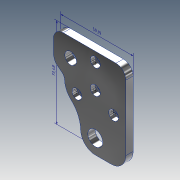
# Autodesk Inventor part: ZBaringBracket
Saved by Autodesk Inventor 2019 (Build 230136000, 136)
## iProperties
Created: 2018-10-14
Part Number: ZBaringBracket
Material: Aluminum 6061
Document SubType Name: Modeling
Designer: LillaHunden
Density: 2.7 g/cm^3
Appearance: Aluminum - Flat
Mass: 59.817 g
Surface Area: 75.5547 cm^2
Volume: 22.1545 cm^3
Author: LillaHunden
Autodesk Inventor part; units mm, degrees
ref_plane "YZ Plane" through (0, 0, 0) normal (1, 0, 0) x (0, 1, 0)
ref_plane "XZ Plane" through (0, 0, 0) normal (0, 1, 0) x (-1, 0, 0)
ref_plane "XY Plane" through (0, 0, 0) normal (0, 0, 1) x (1, 0, 0)
sketch "Sketch1" plane through (0, 0, 0) normal (0, 0, 1) x (1, 0, 0)
  line L0 (6, -5.5) -> (6, -7.5) construction
  line L1 (6, -7.5) -> (25, -7.5) construction
  line L2 (25, -7.5) -> (25, 7.5) construction
  line L3 (25, 7.5) -> (7.55, 7.5) construction
  line L4 (7.55, 7.5) -> (7.55, 2.5) construction
  line L5 (7.55, 2.5) -> (-7.55, 2.5) construction
  line L6 (-7.55, 2.5) -> (-7.55, 7.5) construction
  line L7 (-7.55, 7.5) -> (-25, 7.5) construction
  line L8 (-25, 7.5) -> (-25, -7.5) construction
  line L9 (-25, -7.5) -> (-6, -7.5) construction
  line L10 (-6, -7.5) -> (-6, -5.5) construction
  line L11 (-6, -5.5) -> (6, -5.5) construction
  line L12 (-7.45, 15.5) -> (7.55, 15.5) construction
  line L13 (-7.45, 2.5) -> (-7.45, 15.5) construction
  line L14 (7.55, 2.5) -> (-7.45, 2.5) construction
  line L15 (7.55, 2.5) -> (7.55, 15.5) construction
  line L16 (25, -7.5) -> (-34.185, -7.5)
  line L17 (-34.185, -7.5) -> (-34.185, 35.7282)
  line L18 (-34.185, 35.7282) -> (25, 35.7282)
  line L19 (25, 35.7282) -> (25, -7.5)
  circle A0 centre (15, 0) radius 1.621 projected
  circle A1 centre (-15, 0) radius 1.621 projected
  point P0 (0, 0)
  constraints: 8 end point, 2 parallel, 1 horizontal, 1 perpendicular, 1 point on line
extrude "Extrusion1" add sketch "Sketch1" along normal blind 6 contours L16 L17 L18 L19 | A0 | A1
sketch "Sketch8" plane through (0, 0, 6) normal (0, 0, 1) x (1, 0, 0)
  line L0 (-25, 7.5) -> (-25, -7.5) construction
  line L1 (-7.55, 7.5) -> (-25, 7.5) construction
  circle A0 centre (-20.1, 20.7) radius 5.5 construction
  line L2 (-34.185, -7.5) -> (-34.185, 35.7282) projected
  line L3 (-34.185, 14.1141) -> (-25, 0)
  line L4 (-25, -7.5) -> (-25, 0)
  line L5 (-34.185, 14.1141) -> (-34.185, 26.4425)
  line L6 (-34.185, 35.7282) -> (25, 35.7282) projected
  line L7 (-34.185, -7.5) -> (25, -7.5) projected
  point P0 (0, 0)
  constraints: 6 end point, 2 midpoint, 1 collinear, 1 point on line
extrude "Extrusion4" cut sketch "Sketch8" against normal through all
fillet "Fillet1" radius 3 1 edges at (-25, 0, 3)
fillet "Fillet2" radius 12 1 edges at (-34.185, 14.1141, 3)
fillet "Fillet4" radius 8 1 edges at (-34.185, 35.7282, 3)
fillet "Fillet5" radius 8 1 edges at (25, 35.7282, 3)
sketch "Sketch9" plane through (0, 0, 0) normal (0, 0, -1) x (-1, 0, 0)
  circle A0 centre (20.1, 20.7) radius 4.765
  arc A1 (21.2721, 23.6507) -> (18.4534, 23.4146) centre (20.1, 20.7) ccw projected
  point P0 (0, 0)
  dimension "d32" = 9.53
  constraints: 1 centre point
  measures "d32" diameter of A0
extrude "Extrusion5" cut sketch "Sketch9" against normal blind 3.3
sketch "Sketch10" plane through (-20.1, 20.7, 3.3) normal (0, 0, -1) x (-1, 0, 0)
  circle A0 centre (0, 0) radius 3.25
  point P0 (-20.1, -20.7)
  dimension "d35" = 6.5
  constraints: 1 centre point
  measures "d35" diameter of A0
extrude "Extrusion6" cut sketch "Sketch10" against normal through all
sketch "Sketch11" plane through (25, -7.5, 0) normal (0, -1, 0) x (1, 0, 0)
  line L0 (-50, 6) -> (-50, 0) projected
  line L1 (0, 0) -> (-50, 0) projected
  line L2 (0, 0) -> (0, 6) projected
  line L3 (-50, 6) -> (0, 6) projected
  point P0 (-25, 0)
extrude "Extrusion7" add sketch "Sketch11" along normal blind 30.25
sketch "Sketch12" plane through (0, 0, 6) normal (0, 0, 1) x (1, 0, 0)
  circle A0 centre (0.0605, -25.75) radius 6.1
  line L0 (25, -37.75) -> (-25, -37.75) projected
  point P0 (0, 0)
  dimension "d40" = 12.2
  dimension "d41" = 12
  constraints: 1 centre point
  measures "d40" diameter of A0
  measures "d41" distance from line of A0.centre L0
extrude "Extrusion8" cut sketch "Sketch12" against normal through all
fillet "Fillet6" radius 12 2 edges at (-25, -37.75, 3) (25, -37.75, 3)
sketch "Sketch13" plane through (0, 0, 6) normal (0, 0, 1) x (1, 0, 0)
  line L0 (-25, 5.4183) -> (-25, -8.3317) projected
  arc A0 (-34.185, 17.6749) -> (-32.2428, 11.1296) centre (-22.185, 17.6749) ccw projected
  line L1 (-25, 5.4183) -> (-32.2428, 11.1296)
  line L2 (-32.2428, 11.1296) -> (-25.4856, 0.7461) projected
  arc A1 (-25, -0.8902) -> (-25.4856, 0.7461) centre (-28, -0.8902) ccw projected
  point P0 (0, 0)
  constraints: 2 end point
extrude "Extrusion9" cut sketch "Sketch13" against normal through all
fillet "Fillet7" radius 6 2 edges at (-25, 5.4183, 3) (-32.2428, 11.1296, 3)
sketch "Sketch5" plane through (0, 0, 6) normal (0, 0, 1) x (1, 0, 0)
  point P0 (15, 0)
  point P1 (-15, 0)
sketch "Sketch7" plane through (0, 0, 6) normal (0, 0, 1) x (1, 0, 0)
  point P0 (0.0605, 28)
  point P1 (0.0605, 8)
sketch "Sketch14" plane through (0, 0, 6) normal (0, 0, 1) x (1, 0, 0)
  point P0 (0.0605, 8)
  point P1 (0.0605, 28)
hole "Hole4" at (0.0605, 8, 6) at (0.0605, 28, 6) direction (0, 0, -1) diameter 4.5 depth 6 counterbore diameter 8 counterbore depth 4
sketch "Sketch15" plane through (0, 0, 6) normal (0, 0, 1) x (1, 0, 0)
  point P0 (15, -2.0817)
  point P1 (-15, -2.0817)
hole "Hole6" at (15, -2.0817, 6) at (-15, -2.0817, 6) direction (0, 0, -1) diameter 4.5 depth 6 counterbore diameter 8 counterbore depth 4
sketch "Sketch16" plane through (0, 0, 0) normal (0, 0, -1) x (-1, 0, 0)
  circle A0 centre (20.1, 20.7) radius 4.765 projected
  point P0 (0, 0)
extrude "Extrusion10" cut sketch "Sketch16" against normal through all
sketch "Sketch17" plane through (0, 0, 6) normal (0, 0, 1) x (1, 0, 0)
  circle A0 centre (0.0605, -25.75) radius 6.1 construction
  circle A1 centre (0.0605, -25.75) radius 6.1 construction
  arc A2 (-11.9372, -25.9868) -> (0.0605, -37.75) centre (0.0605, -25.75) ccw
  line L0 (13, -37.75) -> (-13, -37.75) construction
  line L1 (-25, -8.3317) -> (-6.1, -8.3317) construction
  arc A3 (-11.9372, -25.9868) -> (-25, -8.3317) centre (-30.9054, -26.3611) ccw
  circle A4 centre (-20.1, 20.7) radius 4.765 projected
  circle A5 centre (15, -2.0817) radius 4 projected
  circle A6 centre (-15, -2.0817) radius 4 projected
  circle A7 centre (0.0605, 8) radius 4 projected
  circle A8 centre (0.0605, 28) radius 4 projected
  circle A9 centre (0.0605, -25.75) radius 6.1 projected
  arc A10 (-33.0434, 12.5667) -> (-31.3294, 10.4094) centre (-27.6142, 15.1208) ccw projected
  line L2 (-31.3294, 10.4094) -> (-27.2848, 7.22) projected
  arc A11 (-25, 2.5086) -> (-27.2848, 7.22) centre (-31, 2.5086) ccw projected
  line L3 (-25, 2.5086) -> (-25, -25.75) projected
  arc A12 (-25, -25.75) -> (-13, -37.75) centre (-13, -25.75) ccw projected
  line L4 (13, -37.75) -> (-13, -37.75) projected
  arc A13 (13, -37.75) -> (25, -25.75) centre (13, -25.75) ccw projected
  line L5 (25, 27.7282) -> (25, -25.75) projected
  arc A14 (25, 27.7282) -> (17, 35.7282) centre (17, 27.7282) ccw projected
  line L6 (17, 35.7282) -> (-26.185, 35.7282) projected
  arc A15 (-26.185, 35.7282) -> (-34.185, 27.7282) centre (-26.185, 27.7282) ccw projected
  line L7 (-34.185, 27.7282) -> (-34.185, 17.6749) projected
  arc A16 (-34.185, 17.6749) -> (-33.0434, 12.5667) centre (-22.185, 17.6749) ccw projected
  line L8 (0.0605, -37.75) -> (-13, -37.75)
  line L9 (-25, 2.5086) -> (-25, -25.75) projected
  line L10 (-25, 2.5086) -> (-25, -25.75)
  arc A17 (-25, -25.75) -> (-13, -37.75) centre (-13, -25.75) ccw
  point P0 (0, 0)
  constraints: 6 point on circle, 4 end point, 4 tangent, 3 centre point, 1 coincident, 1 horizontal, 1 point on line, 1 vertical
extrude "Extrusion11" cut sketch "Sketch17" against normal through all contours A2 L4 A12 L3 A3
body "Solid1"
